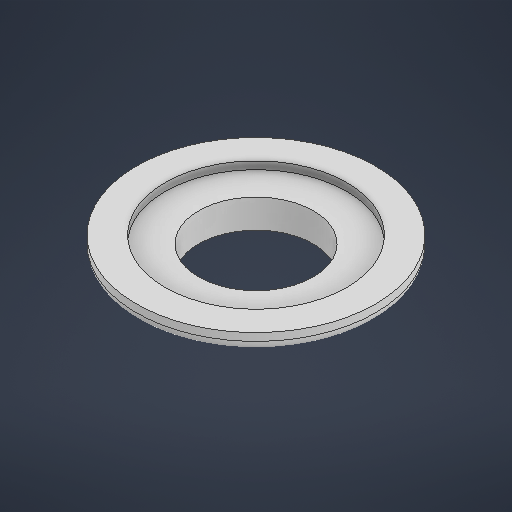
# Autodesk Inventor part: tarcza sprzęgła 2
Saved by Autodesk Inventor 2026.1 (Build 301233020, 233B)
## iProperties
Created: 2026-03-16
Part Number: tarcza sprzęgła 2
Material: Generic
Document SubType Name: Modeling
Designer: Jan
Density: 1 g/cm^3
Appearance: Default
Author: Jan
Autodesk Inventor part; units mm, degrees
ref_plane "YZ Plane" through (0, 0, 0) normal (1, 0, 0) x (0, 1, 0)
ref_plane "XZ Plane" through (0, 0, 0) normal (0, 1, 0) x (-1, 0, 0)
ref_plane "XY Plane" through (0, 0, 0) normal (0, 0, 1) x (1, 0, 0)
sketch "Sketch1" plane through (0, 0, 0) normal (0, 0, 1) x (1, 0, 0)
  line L0 (6, 1.5) -> (6, -1.5)
  line L1 (8, 0.5) -> (11.5, 0.5)
  line L2 (12.5, 1.5) -> (12.5, 2.3)
  line L3 (12.5, 1.5) -> (11.5, 1.5) construction
  line L4 (11.5, 1.5) -> (11.5, 0.5) construction
  arc A0 (11.5, 0.5) -> (12.5, 1.5) centre (11.5, 1.5) ccw
  line L5 (6, 1.5) -> (9.5, 1.5)
  line L6 (12.5, 2.3) -> (9.5, 2.3)
  line L7 (9.5, 2.3) -> (9.5, 1.5)
  line L8 (8, -0.5) -> (8, 0.5)
  line L9 (8, -1.5) -> (8, -0.5)
  line L10 (0, 0) -> (0, 11.9081) construction
  line L11 (8, -1.5) -> (6, -1.5)
  dimension "d0" = 3
  dimension "d1" = 1.5
  dimension "d2" = 0.8
  dimension "d3" = 1
  dimension "d4" = 1
  dimension "d5" = 3
  dimension "d6" = 6
  dimension "d7" = 0.8
  dimension "d8" = 3.5
  constraints: 24 end point, 5 vertical, 3 horizontal, 3 perpendicular, 2 point on circle, 1 centre point, 1 coincident, 1 parallel, 1 tangent
  measures "d0" distance of L5.start L0.end
  measures "d1" vertical distance of L10.start L5.start
  measures "d2" distance of L3.start L2.end
  measures "d3" distance of L3.start L4.start
  measures "d4" distance of L4.start L1.end
  measures "d5" distance of L2.end L7.start
  measures "d6" distance from line of L0 L10.start
  measures "d7" distance of L7.start L5.end
  measures "d8" distance of L5.start L5.end
revolve "Revolution1" add sketch "Sketch1" angle 360 about axis through (0, 0, 0) along (0, 1, 0)
equation "\"d1\" = 0.5 * d0"
equation "\"d4\" = d3"
body "Solid1"
